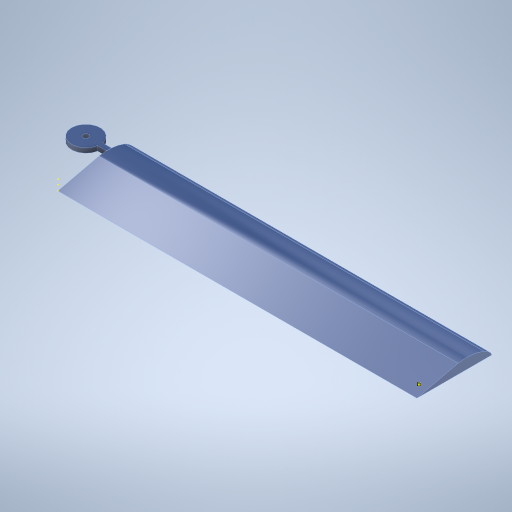
# Autodesk Inventor part: R wing
Saved by Autodesk Inventor 2023 (Build 270158000, 158)
## iProperties
Created: 2023-05-17
Part Number: R wing
Material: Generic
Document SubType Name: Modeling
Designer: Sujeet Kumar
Density: 1 g/cm^3
Appearance: Flaked Satin - Blue
Mass: 830.122 g
Surface Area: 1628.16 cm^2
Volume: 830.122 cm^3
Author: Sujeet Kumar
Autodesk Inventor part; units mm, degrees
ref_plane "YZ Plane" through (0, 0, 0) normal (1, 0, 0) x (0, 1, 0)
ref_plane "XZ Plane" through (0, 0, 0) normal (0, 1, 0) x (-1, 0, 0)
ref_plane "XY Plane" through (0, 0, 0) normal (0, 0, 1) x (1, 0, 0)
sketch "Sketch1" plane through (0, 0, 0) normal (1, 0, 0) x (0, 1, 0)
  line L0 (0, 0) -> (0, -125)
  arc A0 (0, -125) -> (3.9145, -123.4868) centre (-11.1642, -90.2991) ccw
  arc A1 (12.4221, -111.3025) -> (14.7058, -62.5) centre (-60.3675, -83.4416) ccw
  line L1 (0, 0) -> (16.1672, -68.711)
  arc A2 (3.9145, -123.4868) -> (12.4221, -111.3025) centre (-26.7088, -93.042) ccw
  dimension "d0" = 125
  constraints: 7 point on circle, 4 end point, 3 centre point, 1 point on line, 1 vertical
  measures "d0" distance of L0.start L0.end
extrude "Extrusion1" add sketch "Sketch1" along normal blind 600 contours L1 A1 A2 A0 L0
sketch "Sketch2" plane through (0, 0, 0) normal (-1, 0, 0) x (0, 0, 1)
  line L0 (0, 0) -> (-125, 0) projected
  line L1 (-89.759, 17.1606) -> (-81.759, 17.1606)
  line L2 (-81.759, 17.1606) -> (-81.759, 9.1606)
  line L3 (-81.759, 9.1606) -> (-89.759, 9.1606)
  line L4 (-89.759, 9.1606) -> (-89.759, 17.1606)
  line L5 (-89.759, 17.1606) -> (-81.759, 9.1606) construction
  line L6 (-81.759, 17.1606) -> (-89.759, 9.1606) construction
  dimension "d3" = 8
  dimension "d4" = 8
  constraints: 12 end point, 2 parallel, 1 horizontal, 1 perpendicular
  measures "d3" distance of L2.end L3.end
  measures "d4" distance of L1.end L2.end
extrude "Extrusion2" add sketch "Sketch2" along normal blind 48
sketch "Sketch3" plane through (0, 9.1606, -89.759) normal (0, -1, 0) x (1, 0, 0)
  point P0 (0, 89.759)
sketch "Sketch4" plane through (0, 0, 0) normal (0, 0.9734, 0.229) x (1, 0, 0)
  point P0 (0, 0)
sketch "Sketch5" plane through (0, 9.1606, -89.759) normal (0, -1, 0) x (1, 0, 0)
  line L0 (0, 0) -> (-48, 0) projected
  line L1 (0, 0) -> (-39, 0)
  line L2 (-39, 0) -> (-39, 4)
  line L3 (-39, 4) -> (0, 4)
  line L4 (0, 4) -> (0, 0)
  circle A0 centre (-39, 4) radius 24
  circle A1 centre (-39, 4) radius 5
  point P0 (0, 89.759)
  dimension "d7" = 39
  dimension "d8" = 4
  dimension "d9" = 48
  dimension "d12" = 10
  constraints: 8 end point, 2 centre point, 2 coincident, 2 parallel, 1 horizontal, 1 perpendicular
  measures "d7" distance of L2.end L3.end
  measures "d8" distance of L1.end L2.end
  measures "d9" diameter of A0
  measures "d12" diameter of A1
extrude "Extrusion3" add sketch "Sketch5" against normal blind 8 contours A0 L3 A1 L0 | L0 A1 L3 A0 | A1 L0 | L0 L2 L3 A1 | L0 A1 L3 L2
sketch "Sketch6" plane through (0, 17.1606, -81.759) normal (0, 1, 0) x (1, 0, 0)
  point P0 (0, -81.759)
sketch "Sketch7" plane through (0, 9.1606, -89.759) normal (0, -1, 0) x (1, 0, 0)
  point P0 (0, 89.759)
sketch "Sketch8" plane through (0, 9.1606, -89.759) normal (0, -1, 0) x (1, 0, 0)
  line L0 (0, 8) -> (0, 0) projected
  line L1 (0, 0) -> (-39, 0)
  line L2 (-39, 0) -> (-39, 4)
  line L3 (-39, 4) -> (0, 4)
  line L4 (0, 4) -> (0, 0)
  circle A0 centre (-39, 4) radius 5
  point P0 (0, 89.759)
  dimension "d13" = 39
  dimension "d14" = 4
  dimension "d15" = 10
  constraints: 8 end point, 2 parallel, 1 centre point, 1 coincident, 1 horizontal, 1 perpendicular
  measures "d13" distance of L2.end L3.end
  measures "d14" distance of L1.end L2.end
  measures "d15" diameter of A0
extrude "Extrusion4" cut sketch "Sketch8" against normal blind 8 contours A0 L1 L2 L3 | L3 L2 L1 A0
body "Solid1"
